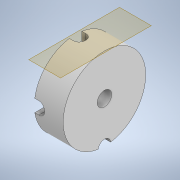
# Autodesk Inventor part: Сердечник
Saved by Autodesk Inventor 2022 (Build 260153000, 153)
## iProperties
Created: 2024-04-28
Part Number: Сердечник
Material: Типовые
Document SubType Name: Modeling
Designer: Pavel
Density: 1 g/cm^3
Appearance: По умолчанию
Author: Pavel
Autodesk Inventor part; units mm, degrees
ref_plane "YZ Plane" through (0, 0, 0) normal (1, 0, 0) x (0, 1, 0)
ref_plane "XY Plane" through (0, 0, 0) normal (0, 0, 1) x (1, 0, 0)
sketch "Эскиз1" plane through (0, 0, 0) normal (0, 1, 0) x (-1, 0, 0)
  line L0 (5.6588, 0) -> (-7.527, 0) construction
  line L1 (0, 0) -> (0, 1.75) construction
  line L2 (0, 1.75) -> (0, 10)
  line L3 (0, 10) -> (7, 10)
  line L4 (7, 10) -> (7, 8)
  line L5 (7, 8) -> (2, 8)
  line L6 (2, 8) -> (2, 3.75)
  line L7 (2, 3.75) -> (7, 3.75)
  line L8 (7, 3.75) -> (7, 1.75)
  line L9 (7, 1.75) -> (0, 1.75)
  dimension "d0" = 1.75
  dimension "d1" = 8.25
  dimension "d2" = 7
  dimension "d3" = 2
  dimension "d4" = 5
  dimension "d5" = 4.25
  dimension "d6" = 2
  constraints: 20 end point, 5 perpendicular, 3 vertical, 1 horizontal
  measures "d0" distance of L1.start L1.end
  measures "d1" distance of L1.end L2.end
  measures "d2" distance of L2.end L3.end
  measures "d3" distance of L3.end L4.end
  measures "d4" distance of L4.end L5.end
  measures "d5" distance of L5.end L6.end
  measures "d6" distance of L7.end L8.end
revolve "Вращение1" add sketch "Эскиз1" angle 360 about axis through (-5.6588, 0, 0) along (1, 0, 0)
ref_plane "РабПлоскость1" through (0, 10, 0) normal (0, 1, 0) x (-1, 0, 0)
sketch "Эскиз3" plane through (0, 10, 0) normal (0, 1, 0) x (-1, 0, 0)
  line L0 (7, -3.75) -> (7, 3.75) construction
  line L1 (7, 0) -> (7, 1.5) construction
  line L2 (7, 1.5) -> (6, 1.5)
  line L3 (7, 0) -> (7, -1.5) construction
  line L4 (7, -1.5) -> (6, -1.5)
  arc A0 (6, 1.5) -> (6, -1.5) centre (6, 0) ccw
  line L5 (7, 1.5) -> (7, -1.5)
  point P0 (0, 0)
  dimension "d12" = 1.5
  dimension "d13" = 1
  dimension "d14" = 1.5
  dimension "d15" = 1
  constraints: 10 end point, 2 perpendicular, 2 point on circle, 2 point on line, 1 centre point, 1 collinear, 1 midpoint
  measures "d12" distance of L1.start L1.end
  measures "d13" distance of L1.end L2.end
  measures "d14" distance of L1.start L3.end
  measures "d15" distance of L3.end L4.end
extrude "Выдавливание1" cut sketch "Эскиз3" against normal blind 2.5
sketch "Эскиз4" plane through (-7, 0, 0) normal (-1, 0, 0) x (0, 0, 1)
  point P0 (0, 0)
  point P1 (0, 0)
  constraints: 1 coincident
pattern_circular "Круговой массив1" count 2 over 90 about axis through (-3.5, 0, 0) along (-1, 0, 0) of "Выдавливание1"
pattern_circular "Круговой массив2" count 2 over 90 about axis through (-3.5, 0, 0) along (1, 0, 0) of "Выдавливание1"
sketch "Эскиз5" plane through (-7, -1.5, -9.8869) normal (-1, 0, 0) x (0, 0, 1)
  line L0 (9.8869, 1.5) -> (9.8869, -10.507) construction
  arc A0 (0, 0) -> (19.7737, 0) centre (9.8869, 1.5) ccw projected
  arc A1 (11.3838, -8.4049) -> (8.3911, -8.3878) centre (9.8869, -8.5) ccw
  point P0 (11.3826, -8.3875)
  point P1 (8.3911, -8.3875)
  dimension "d24" = 1.5
  constraints: 3 point on circle, 2 end point, 1 centre point, 1 point on line, 1 vertical
  measures "d24" radius of A1
extrude "Выдавливание2" cut sketch "Эскиз5" against normal blind 7
sketch "Эскиз7" plane through (-7, -1.5, -9.8869) normal (-1, 0, 0) x (0, 0, 1)
  circle A0 centre (9.8869, -8.5) radius 3
  point P0 (9.8869, 1.5)
  dimension "d28" = 6
  constraints: 1 centre point
  measures "d28" diameter of A0
extrude "Выдавливание3" add sketch "Эскиз7" against normal blind 7
sketch "Эскиз8" plane through (-7, -1.5, -9.8869) normal (-1, 0, 0) x (0, 0, 1)
  circle A0 centre (9.8869, 1.5) radius 10
  dimension "d31" = 20
  constraints: 1 centre point, 1 coincident
  measures "d31" diameter of A0
extrude "Выдавливание4" cut sketch "Эскиз8" against normal blind 7 keep common part
sketch "Эскиз9" plane through (-7, -1.5, -9.8869) normal (-1, 0, 0) x (0, 0, 1)
  circle A0 centre (9.8869, 1.5) radius 10 projected
  circle A1 centre (9.8869, -8.5) radius 1.5
  point P0 (11.3826, -8.3875)
  point P1 (8.3911, -8.3875)
  dimension "d34" = 3
  constraints: 1 centre point, 2 other
  measures "d34" diameter of A1
extrude "Выдавливание5" cut sketch "Эскиз9" against normal blind 7 contours A1 A0 picked at (9.8869, -7.9917)
